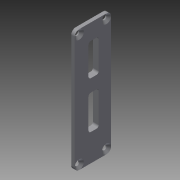
# Autodesk Inventor part: IOModulePlate01
Saved by Autodesk Inventor 2013 (Build 170138000, 138)
## iProperties
Created: 2014-07-14
Part Number: IOModulePlate01
Material: Generic
Document SubType Name: Modeling
Designer: spichelh
Density: 1 g/cm^3
Author: spichelh
Autodesk Inventor part; units mm, degrees
ref_plane "YZ Plane" through (0, 0, 0) normal (1, 0, 0) x (0, 1, 0)
ref_plane "XZ Plane" through (0, 0, 0) normal (0, 1, 0) x (-1, 0, 0)
ref_plane "XY Plane" through (0, 0, 0) normal (0, 0, 1) x (1, 0, 0)
sketch "Sketch1" plane through (0, 0, 0) normal (1, 0, 0) x (0, 1, 0)
  line L0 (2, 0) -> (50.8, 0)
  line L1 (52.8, -2) -> (52.8, -13.8)
  line L2 (50.8, -15.8) -> (2, -15.8)
  line L3 (0, -13.8) -> (0, -2)
  arc A0 (2, 0) -> (0, -2) centre (2, -2) ccw
  arc A1 (0, -13.8) -> (2, -15.8) centre (2, -13.8) ccw
  arc A2 (50.8, -15.8) -> (52.8, -13.8) centre (50.8, -13.8) ccw
  arc A3 (52.8, -2) -> (50.8, 0) centre (50.8, -2) ccw
  circle A4 centre (2, -2) radius 1
  line L4 (26.4, 0) -> (26.4, -6.5481) construction
  line L5 (52.8, -7.9) -> (39.7965, -7.9) construction
  circle A5 centre (50.8, -2) radius 1
  circle A6 centre (2, -13.8) radius 1
  circle A7 centre (50.8, -13.8) radius 1
  point P0 (0, 0)
  point P1 (52.8, 0)
  point P2 (0, -15.8)
  dimension "d0" = 52.8
  dimension "d1" = 15.8
  dimension "d2" = 2
  dimension "d5" = 2
  constraints: 12 end point, 8 centre point, 8 point on circle, 8 tangent, 6 point on line, 3 equal radius, 3 parallel, 3 symmetric about line, 2 midpoint, 2 perpendicular, 1 coincident, 1 horizontal, 3 other
  measures "d0" distance of point (0, 0) point (52.8, 0)
  measures "d1" distance of point (0, -15.8) point (0, 0)
  measures "d2" radius of A0
  measures "d5" diameter of A4
extrude "Extrusion1" add sketch "Sketch1" along normal blind 1.5
chamfer "Chamfer1" distance 1 angle 45 4 edges at (1.5, 49.8, -13.8) (1.5, 49.8, -2) (1.5, 1, -2) (1.5, 1, -13.8)
sketch "Sketch2" plane through (1.5, 0, 0) normal (1, 0, 0) x (0, 0, -1)
  line L0 (0, 50.8) -> (0, 2) projected
  line L1 (7, 45.871) -> (9.4546, 45.871)
  line L2 (10.4546, 44.871) -> (10.4546, 32.8996)
  line L3 (9.4546, 31.8996) -> (7, 31.8996)
  line L4 (6, 32.8996) -> (6, 44.871)
  line L5 (7, 26.5) -> (9.4546, 26.5)
  line L6 (10.4546, 25.5) -> (10.4546, 12.7187)
  line L7 (9.4546, 11.7187) -> (7, 11.7187)
  line L8 (6, 12.7187) -> (6, 25.5)
  arc A0 (10.4546, 44.871) -> (9.4546, 45.871) centre (9.4546, 44.871) ccw
  arc A1 (7, 45.871) -> (6, 44.871) centre (7, 44.871) ccw
  arc A2 (6, 32.8996) -> (7, 31.8996) centre (7, 32.8996) ccw
  arc A3 (9.4546, 31.8996) -> (10.4546, 32.8996) centre (9.4546, 32.8996) ccw
  arc A4 (10.4546, 25.5) -> (9.4546, 26.5) centre (9.4546, 25.5) ccw
  arc A5 (9.4546, 11.7187) -> (10.4546, 12.7187) centre (9.4546, 12.7187) ccw
  arc A6 (6, 12.7187) -> (7, 11.7187) centre (7, 12.7187) ccw
  arc A7 (7, 26.5) -> (6, 25.5) centre (7, 25.5) ccw
  point P0 (0, 0)
  dimension "d9" = 1
  dimension "d10" = 6
  dimension "d11" = 6
  constraints: 16 end point, 16 point on circle, 16 tangent, 8 centre point, 7 equal radius, 4 parallel, 2 horizontal, 2 perpendicular
  measures "d9" radius of A0
  measures "d10" distance between parallel lines of L0 L4
  measures "d11" distance between parallel lines of L0 L8
extrude "Extrusion2" cut sketch "Sketch2" against normal blind 1.5
sketch "Sketch3" plane through (0, 0, 0) normal (-1, 0, 0) x (0, 0, 1)
  arc A0 (-6, 44.871) -> (-7, 45.871) centre (-7, 44.871) ccw projected
  line L0 (-6, 44.871) -> (-6, 32.8996) projected
  arc A1 (-7, 31.8996) -> (-6, 32.8996) centre (-7, 32.8996) ccw projected
  line L1 (-7, 31.8996) -> (-9.4546, 31.8996) projected
  arc A2 (-10.4546, 32.8996) -> (-9.4546, 31.8996) centre (-9.4546, 32.8996) ccw projected
  line L2 (-10.4546, 32.8996) -> (-10.4546, 44.871) projected
  arc A3 (-9.4546, 45.871) -> (-10.4546, 44.871) centre (-9.4546, 44.871) ccw projected
  line L3 (-9.4546, 45.871) -> (-7, 45.871) projected
  arc A4 (-9.4546, 26.5) -> (-10.4546, 25.5) centre (-9.4546, 25.5) ccw projected
  line L4 (-9.4546, 26.5) -> (-7, 26.5) projected
  arc A5 (-6, 25.5) -> (-7, 26.5) centre (-7, 25.5) ccw projected
  line L5 (-6, 25.5) -> (-6, 12.7187) projected
  arc A6 (-7, 11.7187) -> (-6, 12.7187) centre (-7, 12.7187) ccw projected
  line L6 (-7, 11.7187) -> (-9.4546, 11.7187) projected
  arc A7 (-10.4546, 12.7187) -> (-9.4546, 11.7187) centre (-9.4546, 12.7187) ccw projected
  line L7 (-10.4546, 12.7187) -> (-10.4546, 25.5) projected
  line L8 (0, 50.8) -> (0, 2) projected
  line L9 (-13.8, 52.8) -> (-2, 52.8) projected
  line L10 (-12.8, 48.8) -> (-3, 48.8)
  line L11 (-1, 46.8) -> (-1, 6)
  line L12 (-3, 4) -> (-12.8, 4)
  line L13 (-14.8, 6) -> (-14.8, 46.8)
  arc A8 (-12.8, 48.8) -> (-14.8, 46.8) centre (-12.8, 46.8) ccw
  arc A9 (-1, 46.8) -> (-3, 48.8) centre (-3, 46.8) ccw
  arc A10 (-3, 4) -> (-1, 6) centre (-3, 6) ccw
  arc A11 (-14.8, 6) -> (-12.8, 4) centre (-12.8, 6) ccw
  line L14 (-7.9, 52.8) -> (-7.9, 49.069) construction
  line L15 (-7.9, 48.8) -> (-7.9, 44.871) construction
  line L16 (0, 26.4) -> (-3, 26.4) construction
  line L17 (-14.8, 26.4) -> (-12.1303, 26.4) construction
  point P0 (0, 0)
  point P1 (-1, 4)
  point P2 (-1, 48.8)
  point P3 (-14.8, 4)
  dimension "d14" = 13.8
  dimension "d15" = 44.8
  dimension "d16" = 2
  constraints: 16 end point, 8 point on circle, 8 tangent, 6 point on line, 4 centre point, 4 collinear, 4 midpoint, 3 equal radius, 3 perpendicular, 2 parallel, 1 horizontal
  measures "d14" distance of point (-1, 4) point (-14.8, 4)
  measures "d15" distance of point (-1, 48.8) point (-1, 4)
  measures "d16" radius of A8
extrude "Extrusion3" add sketch "Sketch3" along normal blind 1
body "Solid1"
